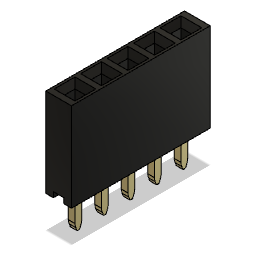
N Pin Female Header 0.1_ (Autodesk Fusion 360 design; units mm, degrees)
Autodesk Fusion 360 part; units mm, degrees
sketch "Sketch11" plane through (0, 0, 0) normal (0, 1, 0) x (1, 0, 0)
  line L0 (1.23, -1.57) -> (-1.23, -1.57)
  line L1 (-1.23, -1.57) -> (-1.23, 11.73)
  line L2 (-1.23, 11.73) -> (1.23, 11.73)
  line L3 (1.23, 11.73) -> (1.23, -1.57)
  dimension "d73" = 2.46
  dimension "d74" = 13.3
  dimension "d78" = 1.23
  dimension "d79" = 1.57
  constraint horizontal L0
  constraint vertical L1
  constraint horizontal L2
  constraint vertical L3
  measures "d73" distance of L0.start L0.end
  measures "d74" distance of L0.start L2.end
  measures "d78" distance of origin L3
  measures "d79" distance of origin L0
extrude "Extrude9" add sketch "Sketch11" along normal blind 8.5 makes body 1
sketch "Sketch12" plane through (0, 8.5, 0) normal (0, 1, 0) x (-1, 0, 0)
  line L0 (-1.23, -11.73) -> (1.23, -11.73)
  line L1 (1.23, -11.73) -> (1.23, 1.57)
  line L2 (1.23, 1.57) -> (-1.23, 1.57)
  line L3 (-1.23, 1.57) -> (-1.23, -11.73)
  line L4 (0.5, -0.5) -> (-0.5, -0.5)
  line L5 (-0.5, -0.5) -> (-0.5, 0.5)
  line L6 (-0.5, 0.5) -> (0.5, 0.5)
  line L7 (0.5, 0.5) -> (0.5, -0.5)
  line L8 (0.5, -0.5) -> (-0.5, 0.5) construction
  line L9 (-0.5, -0.5) -> (0.5, 0.5) construction
  dimension "d80" = 1
  constraint horizontal L4
  constraint perpendicular L4 L5
  constraint parallel L4 L6
  constraint parallel L5 L7
  constraint coincident L8 origin
  constraint coincident L9 origin
  constraint equal L4 L5
  measures "d80" distance of L4.end L5.end
extrude "Extrude10" cut sketch "Sketch12" against normal blind 5 contours L4 L5 L6 L7 bodies 1
chamfer "Chamfer4" distance 0.5 angle 45 4 edges at (0, 8.5, -0.5) (0.5, 8.5, 0) (0, 8.5, 0.5) (-0.5, 8.5, 0) on bodies 1
sketch "Sketch13" plane through (0, 0, 0) normal (0, 1, 0) x (1, 0, 0)
  line L0 (0.5, -1.57) -> (-0.5, -1.57)
  line L1 (-0.5, -1.57) -> (-0.5, 11.73)
  line L2 (-0.5, 11.73) -> (0.5, 11.73)
  line L3 (0.5, 11.73) -> (0.5, -1.57)
  line L4 (0.5, 0.5) -> (0.5, -0.5) construction
  line L5 (-0.5, -0.5) -> (-0.5, 0.5) construction
  line L6 (1.23, -1.57) -> (-1.23, -1.57)
  line L7 (-1.23, 11.73) -> (1.23, 11.73)
  constraint horizontal L0
  constraint vertical L1
  constraint horizontal L2
  constraint vertical L3
  constraint collinear L1 L5
  constraint collinear L3 L4
  constraint collinear L0 L6
  constraint collinear L2 L7
extrude "Extrude11" cut sketch "Sketch13" along normal blind 0.5 bodies 1
pattern_linear "R-Pattern5" count 1 spacing 2.54 along (-1, 0, 0) of "Extrude11"
sketch "Sketch14" plane through (0, 0.5, 0) normal (0, -1, 0) x (1, 0, 0)
  line L0 (0.5, 1.57) -> (-0.5, 1.57)
  line L1 (-0.5, 1.57) -> (-0.5, -11.73)
  line L2 (-0.5, -11.73) -> (0.5, -11.73)
  line L3 (0.5, -11.73) -> (0.5, 1.57)
  line L4 (-0.32, 0.95) -> (0.32, 0.95)
  line L5 (0.32, 0.95) -> (0.32, -0.95)
  line L6 (0.32, -0.95) -> (-0.32, -0.95)
  line L7 (-0.32, -0.95) -> (-0.32, 0.95)
  line L8 (-0.32, 0.95) -> (0.32, -0.95) construction
  line L9 (0.32, 0.95) -> (-0.32, -0.95) construction
  dimension "d93" = 0.64
  dimension "d94" = 1.9
  constraint horizontal L4
  constraint perpendicular L4 L5
  constraint parallel L4 L6
  constraint parallel L5 L7
  constraint coincident L8 origin
  constraint coincident L9 origin
  measures "d93" distance of L5.end L6.end
  measures "d94" distance of L4.end L5.end
extrude "Extrude12" add sketch "Sketch14" along normal blind 0.05 separate body contours L4 L5 L6 L7 makes body 2
sketch "Sketch15" plane through (0, 0.45, 0) normal (0, -1, 0) x (1, 0, 0)
  line L0 (-0.32, -0.95) -> (0.32, -0.95)
  line L1 (0.32, -0.95) -> (0.32, 0.95)
  line L2 (0.32, 0.95) -> (-0.32, 0.95)
  line L3 (-0.32, 0.95) -> (-0.32, -0.95)
  line L4 (-0.32, 0.32) -> (0.32, 0.32)
  line L5 (0.32, 0.32) -> (0.32, -0.32)
  line L6 (0.32, -0.32) -> (-0.32, -0.32)
  line L7 (-0.32, -0.32) -> (-0.32, 0.32)
  line L8 (-0.32, 0.32) -> (0.32, -0.32) construction
  line L9 (0.32, 0.32) -> (-0.32, -0.32) construction
  constraint horizontal L4
  constraint perpendicular L4 L5
  constraint parallel L4 L6
  constraint parallel L5 L7
  constraint coincident L3 L4.start
  constraint coincident L8 origin
  constraint coincident L9 origin
  constraint equal L4 L5
extrude "Extrude13" add sketch "Sketch15" along normal blind 3.5 contours L1 L3 L4 L5 L6 L7 bodies 2
chamfer "Chamfer5" distance 0.2 distance2 0.5 2 edges at (0, -3.05, 0.32) (0, -3.05, -0.32) measured on face at (-0.1067, -3.05, 0.1067) measured on face at (-0.1067, -3.05, 0.1067) on bodies 2
fillet "Fillet2" radius 1 2 edges at (0, -2.55, 0.32) (0, -2.55, -0.32) on bodies 2
pattern_linear "R-Pattern6" count 1 spacing 2.54 along (-1, 0, 0) count 5 spacing 2.54 along (0, 0, -1) of "Extrude10", "Chamfer4"
pattern_linear "R-Pattern7" count 5 spacing 2.54 along (0, 0, -1) of bodies 2 makes body 3 at (0.32, -0.4858, -2.4333) makes body 4 at (-0.32, -0.4858, -5.1867) makes body 5 at (-0.32, -1.4216, -7.5133) makes body 6 at (-0.32, -0.4858, -10.2667)
equation "d73 = ( 2 * 1.23 ) * 1 mm + ( 2.54 * ( Rows - 1 ) ) * 1 mm"
equation "d74 = ( 1.57 * 2 ) * 1 mm + ( 2.54 * ( Columns - 1 ) ) * 1 mm"
equation "Rows = 1"
equation "Columns = 5"
equation "d89 = Rows"
equation "d102 = Rows"
equation "d103 = Columns"
equation "d106 = Columns"
equation "d107 = Rows"
